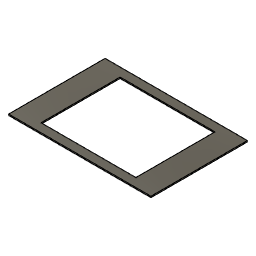
Top Bed v3 (Autodesk Fusion 360 design; units mm, degrees)
Autodesk Fusion 360 part; units mm, degrees
sketch "Sketch1" plane through (0, 0, 0) normal (0, 0, 1) x (1, 0, 0)
  line L0 (-180, 122) -> (180, 122)
  line L1 (180, 122) -> (180, -122)
  line L2 (180, -122) -> (-180, -122)
  line L3 (-180, -122) -> (-180, 122)
  line L4 (-180, 122) -> (180, -122) construction
  line L5 (180, 122) -> (-180, -122) construction
  line L6 (-150, 100) -> (150, 100)
  line L7 (150, 100) -> (150, -100)
  line L8 (150, -100) -> (-150, -100)
  line L9 (-150, -100) -> (-150, 100)
  line L10 (-150, 100) -> (150, -100) construction
  line L11 (150, 100) -> (-150, -100) construction
  dimension "d1" = 244
  dimension "d2" = 360
  dimension "d3" = 300
  dimension "d4" = 200
  constraint horizontal L0
  constraint perpendicular L0 L1
  constraint parallel L0 L2
  constraint parallel L1 L3
  constraint coincident L4 origin
  constraint coincident L5 origin
  constraint horizontal L6
  constraint perpendicular L6 L7
  constraint parallel L6 L8
  constraint parallel L7 L9
  constraint coincident L10 origin
  constraint coincident L11 origin
  measures "d1" distance of L0.end L1.end
  measures "d2" distance of L1 L3
  measures "d3" distance of L7.end L8.end
  measures "d4" distance of L6.end L7.end
extrude "Extrude1" add sketch "Sketch1" along normal blind 3
extrude "Extrude2" add 1 faces at (-150, -33.3333, 1) along direction (1, 0, 0) blind 30
extrude "Extrude3" add 1 faces at (150, 33.3333, 1) along direction (-1, 0, 0) blind 30
sketch "Sketch2" plane through (0, 0, 3) normal (0, 0, 1) x (-1, 0, 0)
  line L0 (-120, 100) -> (120, 100)
  line L1 (120, 100) -> (120, -100)
  line L2 (120, -100) -> (-120, -100)
  line L3 (-120, -100) -> (-120, 100)
  line L4 (180, 122) -> (-180, 122)
  line L5 (-180, 122) -> (-180, -122)
  line L6 (-180, -122) -> (180, -122)
  line L7 (180, -122) -> (180, 122)
